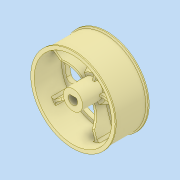
# Autodesk Inventor part: 车轮设计1
Saved by Autodesk Inventor 2019 (Build 230136000, 136)
## iProperties
Created: 2020-10-29
Part Number: 车轮设计1
Material: 尼龙 6/6
Document SubType Name: Modeling
Designer: Wang Hua
Density: 1.13 g/cm^3
Appearance: 尼龙 6
Author: Wang Hua
Autodesk Inventor part; units mm, degrees
ref_plane "YZ Plane" through (0, 0, 0) normal (1, 0, 0) x (0, 1, 0)
ref_plane "XZ Plane" through (0, 0, 0) normal (0, 1, 0) x (-1, 0, 0)
ref_plane "XY Plane" through (0, 0, 0) normal (0, 0, 1) x (1, 0, 0)
sketch "草图1" plane through (0, 0, 0) normal (0, 0, 1) x (1, 0, 0)
  circle A0 centre (0, 0) radius 17
  line L0 (7.8746, 3.2) -> (15.4137, 1.6337)
  line L1 (0, 0) -> (21.7118, 0) construction
  line L2 (7.8746, -3.2) -> (15.4137, -1.6337)
  line L3 (-0.61, 8.4781) -> (3.2093, 15.1641)
  line L4 (5.4768, 6.5004) -> (6.3169, 14.1544)
  line L5 (-8.2516, 2.0397) -> (-13.4302, 7.7382)
  line L6 (-4.4898, 7.2175) -> (-11.5096, 10.3816)
  line L7 (-4.4898, -7.2175) -> (-11.5096, -10.3816)
  line L8 (-8.2516, -2.0397) -> (-13.4302, -7.7382)
  line L9 (5.4768, -6.5004) -> (6.3169, -14.1544)
  line L10 (-0.61, -8.4781) -> (3.2093, -15.1641)
  arc A1 (5.4768, 6.5004) -> (7.8746, 3.2) centre (9.624, 6.9923) ccw
  arc A2 (-4.4898, 7.2175) -> (-0.61, 8.4781) centre (-3.6761, 11.3137) ccw
  arc A3 (-8.2516, -2.0397) -> (-8.2516, 2.0397) centre (-11.896, 0) ccw
  arc A4 (-0.61, -8.4781) -> (-4.4898, -7.2175) centre (-3.6761, -11.3137) ccw
  arc A5 (7.8746, -3.2) -> (5.4768, -6.5004) centre (9.624, -6.9923) ccw
  arc A6 (-7.6128, 3.7809) -> (-8.2516, 2.0397) centre (0, 0) ccw
  arc A7 (3.2093, 15.1641) -> (-11.5096, 10.3816) centre (0, 0) ccw
  arc A8 (-13.4302, 7.7382) -> (-13.4302, -7.7382) centre (0, 0) ccw
  arc A9 (-11.5096, -10.3816) -> (3.2093, -15.1641) centre (0, 0) ccw
  arc A10 (6.3169, -14.1544) -> (15.4137, -1.6337) centre (0, 0) ccw
  arc A11 (15.4137, 1.6337) -> (6.3169, 14.1544) centre (0, 0) ccw
  dimension "d2" = 34
  dimension "d3" = 7.7
  dimension "d4" = 3.2
  dimension "d5" = 21.7118
  dimension "d8" = 360
  dimension "d10" = 4.1763
  dimension "d13" = 360
  dimension "d15" = 8.5
  constraints: 22 end point, 22 point on circle, 12 centre point, 3 coincident, 2 symmetric about line, 1 horizontal, 1 point on line, 52 other
  measures "d2" diameter of A0
  measures "d3" distance of L0.end L0.start
  measures "d4" distance from line of L1 L0.start
  measures "d5" distance of L1.start L1.end
  measures "d10" radius of A1
  measures "d15" radius of A6
extrude "拉伸1" add sketch "草图1" along normal blind 2 contours A0 | L2 A10 L9 A5 | A3 L8 A8 L5 | A4 L10 A9 L7
sketch "草图2" plane through (0, 0, 0) normal (0, 0, -1) x (-1, 0, 0)
  arc A0 (11.5096, 10.3816) -> (-3.2093, 15.1641) centre (0, 0) ccw projected
  line L0 (-3.2093, 15.1641) -> (0.61, 8.4781) projected
  arc A1 (11.5096, 10.3816) -> (-3.2093, 15.1641) centre (0, 0) ccw
  line L1 (-3.2093, 15.1641) -> (0.61, 8.4781)
  line L2 (4.4898, 7.2175) -> (11.5096, 10.3816) projected
  arc A2 (0.61, 8.4781) -> (4.4898, 7.2175) centre (3.6761, 11.3137) ccw
  arc A3 (0.61, 8.4781) -> (4.4898, 7.2175) centre (3.6761, 11.3137) ccw projected
  line L3 (4.4898, 7.2175) -> (11.5096, 10.3816)
  arc A4 (-6.3169, 14.1544) -> (-15.4137, 1.6337) centre (0, 0) ccw
  line L4 (-15.4137, 1.6337) -> (-7.8746, 3.2)
  arc A5 (-7.8746, 3.2) -> (-5.4768, 6.5004) centre (-9.624, 6.9923) ccw
  line L5 (-5.4768, 6.5004) -> (-6.3169, 14.1544)
  arc A6 (-15.4137, -1.6337) -> (-6.3169, -14.1544) centre (0, 0) ccw
  line L6 (-6.3169, -14.1544) -> (-5.4768, -6.5004)
  arc A7 (-5.4768, -6.5004) -> (-7.8746, -3.2) centre (-9.624, -6.9923) ccw
  line L7 (-7.8746, -3.2) -> (-15.4137, -1.6337)
  arc A8 (-3.2093, -15.1641) -> (11.5096, -10.3816) centre (0, 0) ccw
  line L8 (11.5096, -10.3816) -> (4.4898, -7.2175)
  arc A9 (4.4898, -7.2175) -> (0.61, -8.4781) centre (3.6761, -11.3137) ccw
  line L9 (0.61, -8.4781) -> (-3.2093, -15.1641)
  arc A10 (13.4302, -7.7382) -> (13.4302, 7.7382) centre (0, 0) ccw
  line L10 (13.4302, 7.7382) -> (8.2516, 2.0397)
  arc A11 (8.2516, 2.0397) -> (8.2516, -2.0397) centre (11.896, 0) ccw
  line L11 (8.2516, -2.0397) -> (13.4302, -7.7382)
  dimension "d20" = 360
  constraints: 20 end point, 20 point on circle, 10 centre point, 51 other
extrude "拉伸2" cut sketch "草图2" against normal through all contours L7 A7 L6 A6 | L9 A9 L8 A8 | L11 A11 L10 A10
fillet "圆角1" radius 2 10 edges at (3.2093, 15.1641, 1) (15.4137, 1.6337, 1) (6.3169, -14.1544, 1) (-13.4302, 7.7382, 1) (-11.5096, 10.3816, 1) (-13.4302, -7.7382, 1) (-11.5096, -10.3816, 1) (3.2093, -15.1641, 1) (6.3169, 14.1544, 1) (15.4137, -1.6337, 1)
ref_plane "工作平面1" through (0, 0, -1) normal (0, 0, -1) x (-1, 0, 0)
sketch "草图3" plane through (0, 0, -1) normal (0, 0, -1) x (-1, 0, 0)
  circle A0 centre (0, 0) radius 18.5
  circle A1 centre (0, 0) radius 17
  dimension "d26" = 37
  dimension "d29" = 34
  constraints: 2 centre point, 2 coincident
  measures "d26" diameter of A0
  measures "d29" diameter of A1
extrude "拉伸3" add sketch "草图3" against normal blind 15
ref_plane "工作平面2" through (0, 0, 5) normal (0, 0, 1) x (1, 0, 0)
sketch "草图4" plane through (0, 0, 5) normal (0, 0, 1) x (1, 0, 0)
  circle A0 centre (0, 0) radius 5.5
  dimension "d31" = 11
  constraints: 1 centre point, 1 coincident
  measures "d31" diameter of A0
sketch "草图5" plane through (0, 0, 2) normal (0, 0, 1) x (1, 0, 0)
  circle A0 centre (0, 0) radius 7
  dimension "d32" = 14
  constraints: 1 centre point, 1 coincident
  measures "d32" diameter of A0
loft "放样1" add profiles "草图5", "草图4"
sketch "草图6" plane through (0, 0, 5) normal (0, 0, 1) x (1, 0, 0)
  circle A0 centre (0, 0) radius 4.25
  dimension "d37" = 8.5
  constraints: 1 centre point, 1 coincident
  measures "d37" diameter of A0
extrude "拉伸4" add sketch "草图6" along normal up to surface (9 mm away) from surface at 0
sketch "草图7" plane through (0, 0, 14) normal (0, 0, 1) x (1, 0, 0)
  arc A0 (-1.4465, 1.4171) -> (1.4465, 1.4171) centre (0, 0) ccw
  line L0 (1.4465, 1.4171) -> (-1.4465, 1.4171)
  line L1 (-25.9, 0) -> (25.9, 0) projected
  dimension "d40" = 4.05
  dimension "d41" = 2.893
  constraints: 2 end point, 2 point on circle, 1 centre point, 1 coincident, 1 horizontal, 1 parallel
  measures "d40" diameter of A0
  measures "d41" distance of L0.start L0.end
extrude "拉伸5" cut sketch "草图7" against normal blind 8
sketch "草图8" plane through (0, 0, 0) normal (0, 1, 0) x (-1, 0, 0)
  line L0 (-5.5, 5) -> (5.5, 5) construction
  line L1 (-5.5, 5) -> (-7, 2) construction
  line L2 (-7, 2) -> (-5.5, 5) construction
  line L3 (17, 2) -> (-17, 2) projected
  line L4 (-17, 2) -> (-7, 2)
  line L5 (-4.25, 5) -> (4.25, 5) projected
  line L6 (-5.5, 5) -> (-4.25, 5)
  line L7 (-4.25, 5) -> (-4.25, 6.4224)
  line L8 (-4.25, 5) -> (-4.25, 14) projected
  line L9 (-17, 2) -> (-17, 8.875)
  line L10 (-17, 2) -> (-17, 14) projected
  line L11 (-17, 8.875) -> (-12.5502, 8.875)
  arc A0 (-12.5502, 8.875) -> (-4.25, 6.4224) centre (-5.652, 16.9491) ccw
  line L12 (-7, 2) -> (-5.5, 5)
  point P0 (0, 0)
  constraints: 14 end point, 3 point on line, 2 horizontal, 2 point on circle, 1 centre point, 1 collinear
extrude "拉伸6" add sketch "草图8" along normal mid plane 1
pattern_circular "环形阵列1" count 5 over 360 about axis through (0, 0, -10) along (0, 0, 1) of "拉伸6"
fillet "圆角2" radius 1 2 edges at (16.9926, 0.5, 5.4375) (16.9926, -0.5, 5.4375)
pattern_circular "环形阵列2" count 5 over 360 about axis through (0, 0, -10) along (0, 0, 1) of "圆角2"
ref_plane "工作平面3" through (0, 0, 6.5) normal (0, 0, 1) x (1, 0, 0)
ref_plane "工作平面4" through (0, 0, 6.5) normal (0, 0, 1) x (1, 0, 0)
sketch "草图10" plane through (0, 0, 6.5) normal (0, 0, 1) x (1, 0, 0)
  circle A0 centre (0, 0) radius 18.5
  circle A1 centre (0, 0) radius 18
  dimension "d58" = 37
  dimension "d59" = 36
  constraints: 2 centre point, 2 coincident
  measures "d58" diameter of A0
  measures "d59" diameter of A1
extrude "拉伸8" cut sketch "草图10" along normal mid plane 13
fillet "圆角4" radius 0.5 2 edges at (18.5, 0, 0) (18.5, 0, 13)
